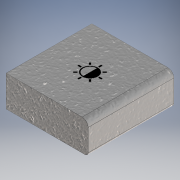
# Autodesk Inventor part: PRZYCISK IO
Saved by Autodesk Inventor 2017 SP1 (Build 210196100, 196)
## iProperties
Created: 2021-03-07
Part Number: PRZYCISK IO
Material: Tworzywo sztuczne, nieprzezroczyste czarne
Document SubType Name: Modeling
Designer: Administrator
Density: 0.952 g/cm^3
Appearance: Teksturowany - szary
Author: Administrator
Autodesk Inventor part; units mm, degrees
ref_plane "YZ Plane" through (0, 0, 0) normal (1, 0, 0) x (0, 1, 0)
ref_plane "XZ Plane" through (0, 0, 0) normal (0, 1, 0) x (-1, 0, 0)
ref_plane "XY Plane" through (0, 0, 0) normal (0, 0, 1) x (1, 0, 0)
sketch "Szkic1" plane through (0, 0, 0) normal (0, 0, 1) x (1, 0, 0)
  line L0 (206.45, -143.65) -> (206.45, -129.275)
  line L1 (206.45, -129.275) -> (220.2, -129.275)
  line L2 (206.45, -143.65) -> (220.2, -143.65)
  line L3 (220.2, -129.275) -> (220.2, -143.65)
  constraints: 8 end point
extrude "Wyciągnięcie proste1" add sketch "Szkic1" against normal blind 5.2
fillet "Zaokrąglenie1" radius 0.5 1 edges at (220.2, -136.4625, -5.2)
sketch "Szkic6" plane through (0, 0, 0) normal (0, 0, 1) x (1, 0, 0)
  arc A0 (213.325, -135.3377) -> (213.325, -137.5873) centre (213.325, -136.4625) ccw
  circle A1 centre (213.325, -136.4625) radius 1.3125
  line L0 (213.4625, -134.4622) -> (213.1875, -134.4622)
  line L1 (213.1875, -134.4622) -> (213.1875, -134.9872)
  line L2 (213.1875, -134.9872) -> (213.4625, -134.9872)
  line L3 (213.4625, -134.9872) -> (213.4625, -134.4622)
  line L4 (210.4962, -136.4625) -> (213.325, -133.6337) construction
  line L5 (212.0078, -134.9509) -> (211.8134, -135.1453)
  line L6 (211.8134, -135.1453) -> (212.1846, -135.5166)
  line L7 (212.1846, -135.5166) -> (212.3791, -135.3221)
  line L8 (212.3791, -135.3221) -> (212.0078, -134.9509)
  line L9 (211.3247, -138.4628) -> (211.3247, -134.4622) construction
  line L10 (211.3247, -136.325) -> (211.3247, -136.6)
  line L11 (211.3247, -136.6) -> (211.8497, -136.6)
  line L12 (211.8497, -136.6) -> (211.8497, -136.325)
  line L13 (211.8497, -136.325) -> (211.3247, -136.325)
  line L14 (213.325, -139.2913) -> (210.4962, -136.4625) construction
  line L15 (211.8134, -137.7797) -> (212.0078, -137.9741)
  line L16 (212.0078, -137.9741) -> (212.3791, -137.6029)
  line L17 (212.3791, -137.6029) -> (212.1846, -137.4084)
  line L18 (212.1846, -137.4084) -> (211.8134, -137.7797)
  line L19 (215.3253, -138.4628) -> (211.3247, -138.4628) construction
  line L20 (213.1875, -138.4628) -> (213.4625, -138.4628)
  line L21 (213.4625, -138.4628) -> (213.4625, -137.9378)
  line L22 (213.4625, -137.9378) -> (213.1875, -137.9378)
  line L23 (213.1875, -137.9378) -> (213.1875, -138.4628)
  line L24 (216.1538, -136.4625) -> (213.325, -139.2913) construction
  line L25 (214.6422, -137.9741) -> (214.8366, -137.7797)
  line L26 (214.8366, -137.7797) -> (214.4654, -137.4084)
  line L27 (214.4654, -137.4084) -> (214.2709, -137.6029)
  line L28 (214.2709, -137.6029) -> (214.6422, -137.9741)
  line L29 (215.3253, -134.4622) -> (215.3253, -138.4628) construction
  line L30 (215.3253, -136.6) -> (215.3253, -136.325)
  line L31 (215.3253, -136.325) -> (214.8003, -136.325)
  line L32 (214.8003, -136.325) -> (214.8003, -136.6)
  line L33 (214.8003, -136.6) -> (215.3253, -136.6)
  line L34 (213.325, -133.6337) -> (216.1538, -136.4625) construction
  line L35 (214.8366, -135.1453) -> (214.6422, -134.9509)
  line L36 (214.6422, -134.9509) -> (214.2709, -135.3221)
  line L37 (214.2709, -135.3221) -> (214.4654, -135.5166)
  line L38 (214.4654, -135.5166) -> (214.8366, -135.1453)
  line L39 (213.325, -136.4625) -> (213.325, -135.3377)
  line L40 (213.325, -136.4625) -> (213.325, -137.5873)
  point P0 (211.3247, -134.4622)
  point P1 (213.325, -134.7247)
  point P2 (212.0962, -135.2337)
  point P3 (211.5872, -136.4625)
  point P4 (212.0962, -137.6913)
  point P5 (213.325, -138.2003)
  point P6 (214.5538, -137.6913)
  point P7 (215.0628, -136.4625)
  point P8 (214.5538, -135.2337)
  dimension "d55" = 2.625
  dimension "d57" = 0.275
  dimension "d61" = 360
  constraints: 68 end point, 2 centre point, 2 parallel, 2 point on circle, 1 coincident, 1 horizontal, 1 perpendicular, 1 point on line, 1 vertical, 95 other
  measures "d55" diameter of A1
  measures "d57" distance of L2.end L1.end
fillet "Zaokrąglenie2" radius 1 1 edges at (220.2, -136.4625, 0)
extrude "Wyciągnięcie proste5" add sketch "Szkic6" along normal blind 0.001 contours L39 L40 A0 | A1 | L3 L2 L1 L0 | L8 L7 L6 L5 | L13 L12 L11 L10 | L18 L17 L16 L15 | L23 L22 L21 L20 | L28 L27 L26 L25 | L33 L32 L31 L30 | L38 L37 L36 L35
